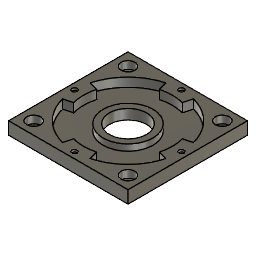
OpenATC-Base-holder (Autodesk Fusion 360 design; units mm, degrees)
Autodesk Fusion 360 part; units mm, degrees
note: some values were not read from the file. Chosen so that the rebuilt part matches the saved one: a direction; a side.
sketch "Sketch1" plane through (0, 0, 0) normal (0, 0, 1) x (1, 0, 0)
  line L0 (-47.5, -47.5) -> (47.5, -47.5)
  line L1 (47.5, -47.5) -> (47.5, 47.5)
  line L2 (47.5, 47.5) -> (-47.5, 47.5)
  line L3 (-47.5, 47.5) -> (-47.5, -47.5)
  line L4 (-37.5, 37.5) -> (-37.5, -37.5) construction
  line L5 (-37.5, -37.5) -> (37.5, -37.5) construction
  line L6 (37.5, 37.5) -> (37.5, -37.5) construction
  line L7 (-37.5, 37.5) -> (-24.7362, 37.5)
  line L8 (-24.7362, 37.5) -> (37.5, 37.5) construction
  line L9 (-47.5, 47.5) -> (47.5, -47.5) construction
  line L10 (-47.5, -47.5) -> (47.5, 47.5) construction
  point P0 (-37.5, 37.5)
  point P1 (37.5, 37.5)
  point P2 (-37.5, -37.5)
  point P3 (37.5, -37.5)
  dimension "d33" = 10
  dimension "d34" = 75
  dimension "d35" = 75
  constraint horizontal L0
  constraint vertical L1
  constraint horizontal L2
  constraint vertical L3
  constraint coincident P0 L4.start
  constraint coincident P2 L4.end
  constraint coincident P3 L5.end
  constraint horizontal L5
  constraint coincident P1 L6.start
  constraint perpendicular L4 L7
  constraint vertical L6
  constraint vertical L4
  constraint horizontal L8
  constraint coincident origin L10
  constraint coincident origin L9
  constraint coincident L0.start L3.end
  constraint coincident P2 L10
  constraint coincident P0 L9
  constraint coincident P1 L10
  measures "d33" distance of L1 L6
  measures "d34" distance of P2 P3
  measures "d35" distance of P0 P2
extrude "Extrude1" add sketch "Sketch1" along normal blind 10
sketch "Sketch2" plane through (0, 0, 10) normal (0, 0, 1) x (-1, 0, 0)
  line L0 (47.5, -47.5) -> (47.5, 47.5)
  line L1 (47.5, 47.5) -> (-47.5, 47.5)
  line L2 (-47.5, 47.5) -> (-47.5, -47.5)
  line L3 (-47.5, -47.5) -> (47.5, -47.5)
  circle A0 centre (0, 0) radius 19.8
  circle A1 centre (0, 0) radius 42.5
  line L4 (0, 0) -> (0, -42.5) construction
  line L5 (10.9998, -41.0518) -> (9.1234, -34.0489)
  line L6 (0, 0) -> (9.1234, -34.0489) construction
  line L7 (0, 0) -> (-9.1234, -34.0489) construction
  line L8 (-9.1234, -34.0489) -> (-10.9998, -41.0518)
  arc A2 (-9.1234, -34.0489) -> (9.1234, -34.0489) centre (0, 0) ccw
  line L9 (41.0518, 10.9998) -> (34.0489, 9.1234)
  arc A3 (34.0489, -9.1234) -> (34.0489, 9.1234) centre (0, 0) ccw
  line L10 (34.0489, -9.1234) -> (41.0518, -10.9998)
  line L11 (-10.9998, 41.0518) -> (-9.1234, 34.0489)
  arc A4 (9.1234, 34.0489) -> (-9.1234, 34.0489) centre (0, 0) ccw
  line L12 (9.1234, 34.0489) -> (10.9998, 41.0518)
  line L13 (-41.0518, -10.9998) -> (-34.0489, -9.1234)
  arc A5 (-34.0489, 9.1234) -> (-34.0489, -9.1234) centre (0, 0) ccw
  line L14 (-34.0489, 9.1234) -> (-41.0518, 10.9998)
  dimension "d9" = 39.6
  dimension "d10" = 85
  dimension "d11" = 35.25
  dimension "d12" = 15
  dimension "d13" = 15
  dimension "d15" = 360
  constraint coincident A0.centre A1.centre
  constraint coincident A1 L4.end
  constraint vertical L4
  constraint coincident A1 L5.start
  constraint coincident A1 L8.end
  constraint parallel L7 L8
  constraint parallel L5 L6
  constraint concentric A1 A2
  measures "d9" diameter of A0
  measures "d10" diameter of A1
  measures "d11" radius of A2
  measures "d12" angle of L4 L5
  measures "d13" angle of L4 L7
extrude "Extrude2" cut sketch "Sketch2" against normal blind 7 contours A1 L5 L8 A2 L9 A3 L10 L11 A4 L12 L13 A5 L14
sketch "Sketch3" plane through (0, 0, 10) normal (0, 0, 1) x (-1, 0, 0)
  circle A0 centre (0, 0) radius 19.8
extrude "Extrude3" cut sketch "Sketch3" against normal up to surface (2 mm away)
sketch "Sketch4" plane through (0, 0, 8) normal (0, 0, 1) x (-1, 0, 0)
  circle A0 centre (0, 0) radius 19.8
  circle A1 centre (0, 0) radius 14.8
  dimension "d36" = 5
  constraint concentric A0 A1
  measures "d36" distance of A0 A1
extrude "Extrude4" cut sketch "Sketch4" against normal through all contours A1
sketch "Sketch6" plane through (0, 0, 10) normal (0, 0, 1) x (-1, 0, 0)
  line L0 (47.5, -47.5) -> (47.5, 47.5)
  line L1 (47.5, 47.5) -> (-47.5, 47.5)
  line L2 (-47.5, 47.5) -> (-47.5, -47.5)
  line L3 (-47.5, -47.5) -> (47.5, -47.5)
  arc A0 (-10.9998, 41.0518) -> (-41.0518, 10.9998) centre (0, 0) ccw
  line L4 (-10.9998, 41.0518) -> (-9.1234, 34.0489)
  arc A1 (9.1234, 34.0489) -> (-9.1234, 34.0489) centre (0, 0) ccw
  line L5 (9.1234, 34.0489) -> (10.9998, 41.0518)
  arc A2 (41.0518, 10.9998) -> (10.9998, 41.0518) centre (0, 0) ccw
  line L6 (41.0518, 10.9998) -> (34.0489, 9.1234)
  arc A3 (34.0489, -9.1234) -> (34.0489, 9.1234) centre (0, 0) ccw
  line L7 (34.0489, -9.1234) -> (41.0518, -10.9998)
  arc A4 (10.9998, -41.0518) -> (41.0518, -10.9998) centre (0, 0) ccw
  line L8 (37.5, -37.5) -> (-37.5, -37.5) construction
  line L9 (-37.5, -37.5) -> (-37.5, 37.5) construction
  line L10 (-37.5, 37.5) -> (37.5, 37.5) construction
  line L11 (37.5, 37.5) -> (37.5, -37.5) construction
  line L12 (-9.1234, -34.0489) -> (-10.9998, -41.0518)
  arc A5 (-41.0518, -10.9998) -> (-10.9998, -41.0518) centre (0, 0) ccw
  line L13 (-41.0518, -10.9998) -> (-34.0489, -9.1234)
  arc A6 (-34.0489, 9.1234) -> (-34.0489, -9.1234) centre (0, 0) ccw
  line L14 (-34.0489, 9.1234) -> (-41.0518, 10.9998)
  line L15 (10.9998, -41.0518) -> (9.1234, -34.0489)
  arc A7 (-9.1234, -34.0489) -> (9.1234, -34.0489) centre (0, 0) ccw
  point P0 (37.5, -37.5)
  point P1 (-37.5, -37.5)
  point P2 (-37.5, 37.5)
  point P3 (37.5, 37.5)
  dimension "d22" = 10
  dimension "d23" = 10
  dimension "d24" = 10
  dimension "d25" = 10
  constraint coincident P0 L8.start
  constraint coincident P1 L8.end
  constraint parallel L3 L8
  constraint coincident P2 L9.end
  constraint perpendicular L3 L9
  constraint coincident P3 L10.end
  constraint perpendicular L9 L10
  constraint vertical L11
  measures "d22" distance of L1 L10
  measures "d23" distance of L0 L11
  measures "d24" distance of L3 L8
  measures "d25" distance of L2 L9
hole "Hole1" at (-37.5, -37.5, 10) at (-37.5, 37.5, 10) at (37.5, 37.5, 10) at (37.5, -37.5, 10) direction (0, 0, -1) diameter 6.6 end through all counterbore diameter 11 counterbore depth 6
sketch "Sketch7" plane through (0, 0, 10) normal (0, 0, 1) x (-1, 0, 0)
  circle A0 centre (-37.5, -37.5) radius 5.5
  circle A1 centre (37.5, 37.5) radius 5.5
  circle A2 centre (37.5, -37.5) radius 5.5
  circle A3 centre (-37.5, 37.5) radius 5.5
  line L0 (47.5, -47.5) -> (47.5, 47.5)
  line L1 (47.5, 47.5) -> (-47.5, 47.5)
  line L2 (-47.5, 47.5) -> (-47.5, -47.5)
  line L3 (-47.5, -47.5) -> (47.5, -47.5)
  line L4 (-9.1234, -34.0489) -> (-10.9998, -41.0518)
  arc A4 (-41.0518, -10.9998) -> (-10.9998, -41.0518) centre (0, 0) ccw
  line L5 (-41.0518, -10.9998) -> (-34.0489, -9.1234)
  arc A5 (-34.0489, 9.1234) -> (-34.0489, -9.1234) centre (0, 0) ccw
  line L6 (-34.0489, 9.1234) -> (-41.0518, 10.9998)
  arc A6 (-10.9998, 41.0518) -> (-41.0518, 10.9998) centre (0, 0) ccw
  line L7 (-10.9998, 41.0518) -> (-9.1234, 34.0489)
  arc A7 (9.1234, 34.0489) -> (-9.1234, 34.0489) centre (0, 0) ccw
  line L8 (9.1234, 34.0489) -> (10.9998, 41.0518)
  arc A8 (41.0518, 10.9998) -> (10.9998, 41.0518) centre (0, 0) ccw
  line L9 (41.0518, 10.9998) -> (34.0489, 9.1234)
  arc A9 (34.0489, -9.1234) -> (34.0489, 9.1234) centre (0, 0) ccw
  line L10 (34.0489, -9.1234) -> (41.0518, -10.9998)
  arc A10 (10.9998, -41.0518) -> (41.0518, -10.9998) centre (0, 0) ccw
  line L11 (10.9998, -41.0518) -> (9.1234, -34.0489)
  arc A11 (-9.1234, -34.0489) -> (9.1234, -34.0489) centre (0, 0) ccw
  line L12 (47.5, 0) -> (-47.5, 0) construction
  line L13 (0, -47.5) -> (0, 47.5) construction
  point P0 (42.5, 0)
  point P1 (-42.5, 0)
  point P2 (0, -42.5)
  point P3 (0, 42.5)
  dimension "d37" = 5
  dimension "d38" = 5
  dimension "d39" = 5
  dimension "d40" = 5
  constraint midpoint L0 L12.start
  constraint midpoint L2 L12.end
  constraint midpoint L3 L13.start
  constraint midpoint L1 L13.end
  constraint coincident L12 P0
  constraint coincident L12 P1
  constraint coincident L13 P2
  constraint coincident L13 P3
  measures "d37" distance of L0 P0
  measures "d38" distance of L1 P3
  measures "d39" distance of L2 P1
  measures "d40" distance of L3 P2
hole "Hole2" at (0, 42.5, 10) at (-42.5, 0, 10) at (0, -42.5, 10) at (42.5, 0, 10) direction (0, 0, -1) diameter 3.332 end through all
thread "Thread1" "ISO Metric profile 4.0 M4x0.7 M4x0.7 6H" thread offset 0 thread depth 7.4
chamfer "Chamfer1" distance 0.4 angle 75 4 edges at (-1.5533, 43.1025, 10) (40.9467, 0.6025, 10) (-1.5533, -41.8975, 10) (-44.0533, 0.6025, 10) measured on face at (-5.2099, -39.359, 10) measured on face at (-5.2099, -39.359, 10) measured on face at (-5.2099, -39.359, 10) measured on face at (-5.2099, -39.359, 10)
equation "d13 = d12"
equation "d23 = d22"
equation "d24 = d22"
equation "d25 = d22"
equation "d35 = d34"
equation "d38 = d37"
equation "d39 = d37"
equation "d40 = d37"
